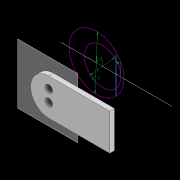
# Autodesk Inventor part: Leaver
Saved by Autodesk Inventor 2022.2 (Build 262287010, 287A)
## iProperties
Created: 2022-06-02
Part Number: Leaver
Material: Generic
Document SubType Name: Modeling
Designer: Árni Þór Þorgeirsson
Density: 1 g/cm^3
Appearance: Default
Author: Árni Þór Þorgeirsson
Autodesk Inventor part; units mm, degrees
ref_plane "YZ Plane" through (0, 0, 0) normal (1, 0, 0) x (0, 1, 0)
ref_plane "XZ Plane" through (0, 0, 0) normal (0, 1, 0) x (-1, 0, 0)
sketch "Sketch1" plane through (0, 0, 0) normal (0, 0, 1) x (1, 0, 0)
  circle A0 centre (0, 0) radius 11.25
  line L0 (0, 0) -> (2.5, 0)
  circle A1 centre (2.5, 0) radius 7.5
  line L1 (8, 6.7455) -> (8, -7.7933)
  point P0 (10, 0)
  point P1 (10, 0)
  point P2 (8, -5.099)
  point P3 (8, 5.099)
  dimension "d2" = 15
  dimension "d0" = 22.5
  dimension "d1" = 2.5
  dimension "d3" = 2
  constraints: 4 end point, 3 coincident, 1 centre point, 1 horizontal, 1 vertical, 3 other
  measures "d0" diameter of A0
  measures "d1" distance of L0.start L0.end
  measures "d3" distance from line of point (10, 0) L1
extrude "Extrusion1" [suppressed]
extrude "Extrusion2" [suppressed]
sketch "Sketch2" plane through (2.5, 0, 13.5) normal (0, 0, 1) x (1, 0, 0)
  line L0 (0, 0) -> (0, 3)
  circle A0 centre (0, 3) radius 2.75
  line L1 (-18.25, 0) -> (13.25, 0) construction
  circle A1 centre (0, -3) radius 2.75
  point P0 (-2.5, 0)
  dimension "d8" = 3
  dimension "d23" = 5.5
  constraints: 2 centre point, 2 end point, 1 coincident, 1 symmetric about line, 1 vertical, 1 other
  measures "d8" distance of L0.start L0.end
  measures "d23" diameter of A0
hole "Hole1" [suppressed]
feature "FaceDraft1" [suppressed]
ref_plane "Work Plane1" through (0, 0, 20) normal (0, 0, 1) x (1, 0, 0)
sketch "Sketch3" plane through (0, 0, 20) normal (0, 0, 1) x (1, 0, 0)
  arc A0 (8, 5.099) -> (8, -5.099) centre (2.5, 0) ccw projected
  circle A1 centre (2.5, 3) radius 1.5 projected
  circle A2 centre (2.5, -1.8526) radius 1.5 projected
  line L0 (2.5, 7.5) -> (27.5, 7.5)
  line L1 (2.5, -7.5) -> (27.5, -7.5)
  line L2 (27.5, -7.5) -> (27.5, 7.5)
  point P0 (0, 0)
  dimension "d18" = 25
  dimension "d19" = 25
  constraints: 6 end point, 2 horizontal, 2 point on circle, 1 perpendicular
  measures "d18" distance of L0.start L0.end
  measures "d19" distance of L1.start L1.end
extrude "Extrusion3" add sketch "Sketch3" along normal blind 2
body "Solid1"
